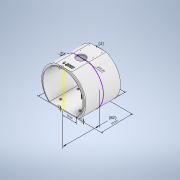
# Autodesk Inventor part: body-3
Saved by Autodesk Inventor 2020 (Build 240168000, 168)
## iProperties
Created: 2019-10-07
Part Number: body-3
Material: ABS Plastic
Document SubType Name: Modeling
Designer: sl65b
Density: 1.06 g/cm^3
Appearance: Smooth - White
Mass: 111.574 g
Surface Area: 610.266 cm^2
Volume: 105.258 cm^3
Author: sl65b
Autodesk Inventor part; units mm, degrees
ref_plane "YZ Plane" through (0, 0, 0) normal (1, 0, 0) x (0, 1, 0)
ref_plane "XY Plane" through (0, 0, 0) normal (0, 0, 1) x (1, 0, 0)
sketch "Sketch1" plane through (0, 0, 0) normal (0, 0, 1) x (1, 0, 0)
  point P0 (0, 0)
sketch "Sketch2" plane through (0, 0, 0) normal (0, 0, 1) x (1, 0, 0)
  line L0 (-17.5, 82.5465) -> (17.5, 82.5465)
  arc A0 (35, 0.0018) -> (17.5, 82.5465) centre (0, 35.709) ccw
  arc A1 (-17.5, 82.5465) -> (-35, 0.0018) centre (0, 35.709) ccw
  line L1 (-35, 0.0018) -> (35, 0.0018)
  line L2 (0, 0) -> (0, 40.607)
  point P0 (-7.6811, -29)
  dimension "d67" = 35
  dimension "d173" = 50
  dimension "d174" = 50
  dimension "d178" = 70
  constraints: 6 end point, 4 point on circle, 2 centre point, 2 vertical, 1 parallel, 1 point on line, 2 other
  measures "d67" distance of L0.start L0.end
  measures "d173" radius of A1
  measures "d174" radius of A0
  measures "d178" distance of L1.start L1.end
sketch "Sketch6" plane through (0, 0, 0) normal (0, 0, 1) x (1, 0, 0)
  arc A0 (30, -0.0205) -> (-30, -0.0205) centre (0, 35.4445) ccw
  line L0 (30, -0.0205) -> (-30, -0.0205)
  line L1 (0, 0) -> (0, 43.5003)
  line L2 (0, 0) -> (40.6393, 0)
  point P0 (0, 32.4176)
  dimension "d171" = 60
  constraints: 6 end point, 2 horizontal, 2 point on circle, 2 vertical, 1 centre point, 1 point on line
  measures "d171" distance of L0.end L0.start
extrude "Extrusion1" add sketch "Sketch6" along normal mid plane 82
extrude "Extrusion2" add sketch "Sketch2" along normal mid plane 78
sketch "Sketch25" plane through (0, 0, 0) normal (1, 0, 0) x (0, 1, 0)
  line L0 (0.0018, -39) -> (82.5465, -39) projected
  line L1 (-0.0205, -41) -> (81.8962, -41) projected
  line L2 (82.5465, 39) -> (0.0018, 39) projected
  line L3 (81.8962, 41) -> (-0.0205, 41) projected
  point P0 (0, 0)
  dimension "d64" = 2
  dimension "d65" = 2
  measures "d64" distance between parallel lines of L0 L1
  measures "d65" distance between parallel lines of L2 L3
sketch "Sketch26" plane through (0, 0, 0) normal (1, 0, 0) x (0, 1, 0)
  line L0 (-0.0205, -41) -> (81.8962, -41) projected
  line L1 (81.8962, 41) -> (-0.0205, 41) projected
  point P0 (0, 0)
  dimension "d66" = 82
  measures "d66" distance between parallel lines of L0 L1
ref_plane "Work Plane8" through (-17.5, 82.5465, -39) normal (0, 1, 0) x (-1, 0, 0)
sketch "Sketch27" plane through (-17.5, 82.5465, -39) normal (0, 1, 0) x (-1, 0, 0)
  circle A0 centre (-17.5, 39) radius 10
  dimension "d69" = 20
  constraints: 1 centre point, 1 coincident
  measures "d69" diameter of A0
extrude "Extrusion8" cut sketch "Sketch27" against normal blind 9.25
sketch "Sketch29" plane through (-17.5, 82.5465, -39) normal (0, 1, 0) x (-1, 0, 0)
  line L0 (-29.6285, 71.2778) -> (-3.5559, 71.2778) construction
  line L1 (-3.5559, 71.2778) -> (-3.5559, 64.4303) construction
  line L2 (-3.5559, 64.4303) -> (-29.6285, 64.4303) construction
  line L3 (-29.6285, 64.4303) -> (-29.6285, 71.2778) construction
  line L4 (-28.3224, 68.6656) -> (-28.3224, 65.1778)
  line L5 (-28.3224, 65.1778) -> (-29.6285, 65.1778)
  line L6 (-29.6285, 65.1778) -> (-29.6285, 71.2778)
  line L7 (-29.6285, 71.2778) -> (-28.3224, 71.2778)
  line L8 (-28.3224, 71.2778) -> (-27.6669, 69.7516)
  line L9 (-27.6669, 69.7516) -> (-27.0163, 71.2778)
  line L10 (-27.0163, 71.2778) -> (-25.7054, 71.2778)
  line L11 (-25.7054, 71.2778) -> (-25.7054, 65.1778)
  line L12 (-25.7054, 65.1778) -> (-27.0163, 65.1778)
  line L13 (-27.0163, 65.1778) -> (-27.0163, 68.6656)
  line L14 (-27.0163, 68.6656) -> (-27.6669, 67.3547)
  line L15 (-27.6669, 67.3547) -> (-28.3224, 68.6656)
  spline S0 degree 2 poles (-23.0981, 71.2778) (-22.2273, 71.2778) (-21.792, 70.8425) knots 0 0 0 1 1 1
  line L16 (-21.792, 70.8425) -> (-21.792, 65.1778)
  line L17 (-21.792, 65.1778) -> (-23.0981, 65.1778)
  line L18 (-23.0981, 65.1778) -> (-23.0981, 67.79)
  line L19 (-23.0981, 67.79) -> (-23.5334, 67.79)
  line L20 (-23.5334, 67.79) -> (-23.5334, 65.1778)
  line L21 (-23.5334, 65.1778) -> (-24.8395, 65.1778)
  line L22 (-24.8395, 65.1778) -> (-24.8395, 70.8425)
  spline S1 degree 2 poles (-24.8395, 70.8425) (-24.4042, 71.2778) (-23.5334, 71.2778) knots 0 0 0 1 1 1
  line L23 (-23.5334, 71.2778) -> (-23.0981, 71.2778)
  line L24 (-23.5334, 70.4071) -> (-23.5334, 68.6656)
  line L25 (-23.5334, 68.6656) -> (-23.0981, 68.6656)
  line L26 (-23.0981, 68.6656) -> (-23.0981, 70.4071)
  line L27 (-23.0981, 70.4071) -> (-23.5334, 70.4071)
  spline S2 degree 2 poles (-19.1798, 71.2778) (-18.309, 71.2778) (-17.8737, 70.8425) knots 0 0 0 1 1 1
  line L28 (-17.8737, 70.8425) -> (-17.8737, 68.6656)
  spline S3 degree 2 poles (-17.8737, 68.6656) (-17.8737, 68.3575) (-18.5243, 68.2254) knots 0 0 0 1 1 1
  spline S4 degree 2 poles (-18.5243, 68.2254) (-17.8737, 68.0982) (-17.8737, 67.79) knots 0 0 0 1 1 1
  line L29 (-17.8737, 67.79) -> (-17.8737, 65.1778)
  line L30 (-17.8737, 65.1778) -> (-19.1798, 65.1778)
  line L31 (-19.1798, 65.1778) -> (-19.1798, 67.79)
  line L32 (-19.1798, 67.79) -> (-19.6151, 67.79)
  line L33 (-19.6151, 67.79) -> (-19.6151, 65.1778)
  line L34 (-19.6151, 65.1778) -> (-20.9212, 65.1778)
  line L35 (-20.9212, 65.1778) -> (-20.9212, 71.2778)
  line L36 (-20.9212, 71.2778) -> (-19.1798, 71.2778)
  line L37 (-19.6151, 70.4071) -> (-19.6151, 68.6656)
  line L38 (-19.6151, 68.6656) -> (-19.1798, 68.6656)
  line L39 (-19.1798, 68.6656) -> (-19.1798, 70.4071)
  line L40 (-19.1798, 70.4071) -> (-19.6151, 70.4071)
  line L41 (-15.6969, 65.1778) -> (-17.003, 65.1778)
  line L42 (-17.003, 65.1778) -> (-17.003, 71.2778)
  line L43 (-17.003, 71.2778) -> (-15.6969, 71.2778)
  line L44 (-15.6969, 71.2778) -> (-15.6969, 68.6656)
  line L45 (-15.6969, 68.6656) -> (-15.2615, 68.6656)
  line L46 (-15.2615, 68.6656) -> (-15.2615, 71.2778)
  line L47 (-15.2615, 71.2778) -> (-13.9554, 71.2778)
  line L48 (-13.9554, 71.2778) -> (-13.9554, 68.6656)
  spline S5 degree 2 poles (-13.9554, 68.6656) (-13.9554, 68.3575) (-14.606, 68.2254) knots 0 0 0 1 1 1
  spline S6 degree 2 poles (-14.606, 68.2254) (-13.9554, 68.0982) (-13.9554, 67.79) knots 0 0 0 1 1 1
  line L49 (-13.9554, 67.79) -> (-13.9554, 65.1778)
  line L50 (-13.9554, 65.1778) -> (-15.2615, 65.1778)
  line L51 (-15.2615, 65.1778) -> (-15.2615, 67.79)
  line L52 (-15.2615, 67.79) -> (-15.6969, 67.79)
  line L53 (-15.6969, 67.79) -> (-15.6969, 65.1778)
  line L54 (-10.4382, 66.9193) -> (-10.4382, 71.2778)
  line L55 (-10.4382, 71.2778) -> (-9.1321, 71.2778)
  line L56 (-9.1321, 71.2778) -> (-9.1321, 67.79)
  line L57 (-9.1321, 67.79) -> (-8.6968, 67.79)
  line L58 (-8.6968, 67.79) -> (-8.6968, 71.2778)
  line L59 (-8.6968, 71.2778) -> (-7.3907, 71.2778)
  line L60 (-7.3907, 71.2778) -> (-7.3907, 65.1778)
  line L61 (-7.3907, 65.1778) -> (-8.6968, 65.1778)
  line L62 (-8.6968, 65.1778) -> (-8.6968, 66.9193)
  line L63 (-8.6968, 66.9193) -> (-10.4382, 66.9193)
  point P0 (-17.5, 39)
  constraints: 2 other
extrude "Extrusion9" add sketch "Sketch29" along normal blind 0.25
sketch "Sketch43" plane through (0, 0, 41) normal (0, 0, 1) x (1, 0, 0)
  point P0 (0, 0)
sketch "Sketch44" plane through (0, 0, -41) normal (0, 0, -1) x (-1, 0, 0)
  point P0 (0, 0)
sketch "Sketch45" plane through (0, 0, 41) normal (0, 0, 1) x (1, 0, 0)
  arc A0 (30, -0.0205) -> (-30, -0.0205) centre (0, 35.4445) ccw projected
  line L0 (-30.0832, 1.9139) -> (30.0832, 1.9139)
  line L1 (-30, 2.9139) -> (30, 2.9139) projected
  arc A1 (30.0832, 1.9139) -> (-30.0832, 1.9139) centre (0, 35.4445) ccw
  point P0 (0, 0)
  dimension "d182" = 1.404
  dimension "d185" = 1
  constraints: 2 end point, 2 point on circle, 1 centre point, 1 coincident, 1 horizontal
  measures "d182" radial gap between concentric circles of A1 A0
  measures "d185" distance between parallel lines of L1 L0
extrude "Extrusion13" cut sketch "Sketch45" against normal blind 69
sketch "Sketch46" plane through (0, 0, -41) normal (0, 0, -1) x (-1, 0, 0)
  arc A0 (30.0832, 1.9139) -> (-30.0832, 1.9139) centre (0, 35.4445) ccw
  line L0 (30, -0.0205) -> (-30, -0.0205) projected
  arc A1 (-30.0832, 1.9139) -> (-27.7766, -0.0205) centre (0, 35.4445) ccw
  arc A2 (27.7766, -0.0205) -> (30.0832, 1.9139) centre (0, 35.4445) ccw
  line L1 (-27.7766, -0.0205) -> (27.7766, -0.0205)
  point P0 (0, 0)
  constraints: 6 point on circle, 3 centre point, 3 point on line, 2 end point
extrude "Extrusion14" cut sketch "Sketch46" against normal blind 11
sketch "Sketch47" plane through (0, 0, -30) normal (0, 0, -1) x (-1, 0, 0)
  line L0 (0, 35.96) -> (-6, 35.96)
  line L1 (0, 35.96) -> (6, 35.96)
  line L2 (6, 35.96) -> (6, 28.66)
  line L3 (6, 28.66) -> (-6, 28.66)
  line L4 (-6, 28.66) -> (-6, 35.96)
  circle A0 centre (-3, 32.31) radius 1.5
  circle A1 centre (3, 32.31) radius 1.5
  point P0 (0, 0)
  dimension "d192" = 35.96
  dimension "d194" = 6
  dimension "d195" = 7.3
  dimension "d196" = 3
  dimension "d197" = 3
  constraints: 10 end point, 3 horizontal, 2 centre point, 2 perpendicular
  measures "d192" distance of point (0, 0) L0.start
  measures "d194" distance of L0.start L1.end
  measures "d195" distance of L1.end L2.end
  measures "d196" diameter of A0
  measures "d197" diameter of A1
extrude "Extrusion15" add sketch "Sketch47" along normal blind 3
sketch "Sketch50" plane through (3, 32.31, -30) normal (0, 0, -1) x (-1, 0, 0)
  circle A0 centre (0, 0) radius 1.5 projected
  line L0 (0, 1.5) -> (0, 0)
  point P0 (3, -32.31)
  constraints: 2 end point, 1 vertical, 1 vertical alignment, 1 other
hole "Hole8" at (3, 32.31, -30) direction (0, 0, 1) diameter 3 depth 10.5 tip angle 118
sketch "Sketch51" plane through (-3, 32.31, -30) normal (0, 0, -1) x (-1, 0, 0)
  circle A0 centre (0, 0) radius 1.5 projected
  line L0 (0, 1.5) -> (0, 0)
  point P0 (-3, -32.31)
  constraints: 2 end point, 1 vertical, 1 vertical alignment, 1 other
hole "Hole9" at (-3, 32.31, -30) direction (0, 0, 1) diameter 3 depth 10.5 tip angle 118
sketch "Sketch53" plane through (0, 0, -39) normal (0, 0, -1) x (-1, 0, 0)
  line L0 (-30.0832, 1.9139) -> (-36.8496, 1.9139)
  line L1 (-30.0264, 0.0018) -> (-35, 0.0018) projected
  line L2 (-27.7766, -0.0205) -> (-35, 0.0018)
  line L3 (30.0832, 1.9139) -> (36.8527, 1.9139)
  line L4 (35, 0.0018) -> (30.0264, 0.0018) projected
  line L5 (27.7766, -0.0205) -> (35, 0.0018)
  arc A0 (27.7766, -0.0205) -> (30.0832, 1.9139) centre (0, 35.4445) ccw
  arc A1 (35, 0.0018) -> (36.8527, 1.9139) centre (-2.4287, 38.1229) ccw
  arc A2 (-36.8496, 1.9139) -> (-35, 0.0018) centre (0, 35.709) ccw
  arc A3 (-30.0832, 1.9139) -> (-27.7766, -0.0205) centre (0, 35.4445) ccw
  point P0 (0, 0)
  constraints: 8 end point, 8 point on circle, 4 centre point, 2 horizontal, 1 point on line
extrude "Extrusion16" add sketch "Sketch53" along normal blind 5
sketch "Sketch54" plane through (0, 0, -44) normal (0, 0, -1) x (-1, 0, 0)
  line L0 (-35, 0.0018) -> (35, 0.0018)
  arc A0 (-36.8496, 1.9139) -> (-35, 0.0018) centre (0, 35.709) ccw
  arc A1 (35, 0.0018) -> (36.8527, 1.9139) centre (-2.4287, 38.1229) ccw
  line L1 (-36.8496, 1.9139) -> (-32.1475, 1.9139) projected
  line L2 (-36.8496, 1.9139) -> (36.8527, 1.9139)
  point P0 (0, 0)
  point P1 (35.92, 0.9274)
  constraints: 5 point on circle, 4 end point, 2 centre point, 1 collinear
extrude "Extrusion18" add sketch "Sketch54" along normal blind 6
sketch "Sketch55" plane through (0, 0, -30) normal (0, 0, -1) x (-1, 0, 0)
  circle A0 centre (0, 67.2827) radius 10
  point P0 (0, 0)
  dimension "d291" = 20
  constraints: 1 centre point
  measures "d291" diameter of A0
hole "Hole10" at (0, 67.2827, -30) direction (0, 0, 1) diameter 15 depth 10.5 tip angle 118
sketch "Sketch56" plane through (-30.0832, 1.9139, 41) normal (0, 1, 0) x (1, 0, 0)
  line L0 (-4.9168, 2) -> (0.0569, 2) projected
  line L1 (0.0569, 2) -> (62.5964, 2)
  line L2 (60.1096, 2) -> (65.0832, 2) projected
  line L3 (30.0832, 2) -> (15.5582, 2)
  line L4 (15.5582, 2) -> (15.5582, 63.6826)
  line L5 (0.5582, 2) -> (0.5582, 63.6826)
  line L6 (0.0569, 2) -> (0.0569, 80) projected
  line L7 (30.0832, 2) -> (44.6082, 2)
  line L8 (44.6082, 2) -> (44.6082, 63.6826)
  line L9 (59.6082, 2) -> (59.6082, 64.3714)
  line L10 (60.0832, 0) -> (60.0832, 82) projected
  circle A0 centre (8.0582, 16.95) radius 1.15
  circle A1 centre (8.0582, 56.75) radius 1.15
  circle A2 centre (52.1082, 16.95) radius 1.15
  circle A3 centre (52.1082, 56.75) radius 1.15
  point P0 (30.0832, 41)
  dimension "d262" = 14.525
  dimension "d263" = 15
  dimension "d264" = 14.525
  dimension "d265" = 15
  dimension "d266" = 2.3
  dimension "d267" = 14.95
  dimension "d268" = 7.5
  dimension "d269" = 2.3
  dimension "d270" = 37.5
  dimension "d271" = 2.3
  dimension "d272" = 7.5
  dimension "d273" = 2.3
  constraints: 14 end point, 5 point on line, 4 centre point, 3 vertical, 1 midpoint, 1 parallel
  measures "d262" distance of L3.start L3.end
  measures "d263" distance between parallel lines of L5 L4
  measures "d264" distance of L3.start L7.end
  measures "d265" distance between parallel lines of L9 L8
  measures "d266" diameter of A0
  measures "d267" distance from line of L1 A0.centre
  measures "d268" distance from line of L4 A0.centre
  measures "d269" diameter of A1
  measures "d271" diameter of A2
  measures "d272" distance from line of L8 A2.centre
  measures "d273" diameter of A3
hole "Hole11" at (-22.025, 1.9139, 24.05) at (-22.025, 1.9139, -15.75) at (22.025, 1.9139, -15.75) at (22.025, 1.9139, 24.05) direction (0, -1, 0) diameter 2.3 depth 15.664 counterbore diameter 5 counterbore depth 0.7
sketch "Sketch57" plane through (-17.5, 82.5465, 39) normal (0, 1, 0) x (1, 0, 0)
  line L0 (63.9517, 78) -> (-28.9517, 78) projected
  line L1 (2, 78) -> (2, 46.6208)
  line L2 (0, 78) -> (0, 0) projected
  line L3 (33, 78) -> (33, 47.9439)
  line L4 (35, 78) -> (35, 0) projected
  line L5 (2, 50.0103) -> (33, 50.0103)
  line L6 (2, 73.5103) -> (33, 73.5103)
  circle A0 centre (3.5, 51.5103) radius 0.5
  circle A1 centre (3.5, 72.0103) radius 0.5
  circle A2 centre (31.5, 51.5103) radius 0.5
  circle A3 centre (31.5, 72.0103) radius 0.5
  point P0 (17.5, 39)
  point P1 (-14.6475, 78)
  point P2 (49.6475, 78)
  dimension "d292" = 2
  dimension "d293" = 2
  dimension "d294" = 23.5
  dimension "d295" = 1
  dimension "d296" = 1.5
  dimension "d297" = 1.5
  dimension "d298" = 1
  dimension "d299" = 1.5
  dimension "d300" = 1
  dimension "d301" = 1.5
  dimension "d302" = 1.5
  dimension "d303" = 1
  constraints: 8 end point, 6 point on line, 4 centre point, 3 perpendicular, 1 horizontal, 1 vertical
  measures "d292" distance between parallel lines of L1 L2
  measures "d293" distance between parallel lines of L4 L3
  measures "d294" distance between parallel lines of L6 L5
  measures "d295" diameter of A0
  measures "d296" distance from line of L1 A0.centre
  measures "d297" distance from line of L5 A0.centre
  measures "d298" diameter of A1
  measures "d299" distance from line of L6 A1.centre
  measures "d300" diameter of A2
  measures "d301" distance from line of L3 A2.centre
  measures "d302" distance from line of L5 A2.centre
  measures "d303" diameter of A3
hole "Hole12" at (-14, 82.5465, -12.5103) at (-14, 82.5465, -33.0103) at (14, 82.5465, -33.0103) at (14, 82.5465, -12.5103) direction (0, -1, 0) diameter 1 depth 10.5 tip angle 118
body "Solid1"
